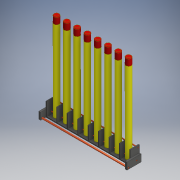
# Autodesk Inventor part: Rampa Lápices 2
Saved by Autodesk Inventor 2016 (Build 200138000, 138)
## iProperties
Created: 2016-06-22
Part Number: Rampa Lápices 2
Material: Generic
Document SubType Name: Modeling
Designer: SCM
Density: 1 g/cm^3
Appearance: Generic
Author: SCM
Autodesk Inventor part; units mm, degrees
ref_plane "YZ Plane" through (0, 0, 0) normal (1, 0, 0) x (0, 1, 0)
sketch "Sketch1" plane through (0, 0, 0) normal (0, 0, 1) x (1, 0, 0)
  line L0 (-120, -20) -> (120, -20)
  line L1 (120, -20) -> (120, 20)
  line L2 (120, 20) -> (-120, 20) construction
  line L3 (-120, 20) -> (-120, -20)
  line L4 (-120, 20) -> (-117.5, 20)
  line L5 (-117.5, 20) -> (-117.5, -17.5)
  line L6 (-117.5, -17.5) -> (117.5, -17.5) construction
  line L7 (117.5, -17.5) -> (117.5, 20)
  line L8 (120, 20) -> (117.5, 20)
  line L9 (-90.3125, -17.5) -> (-87.8125, -17.5) construction
  line L10 (-87.8125, -17.5) -> (-87.8125, 20)
  line L11 (-87.8125, 20) -> (-90.3125, 20)
  line L12 (-90.3125, 20) -> (-90.3125, -17.5)
  line L13 (-60.625, -17.5) -> (-58.125, -17.5) construction
  line L14 (-58.125, -17.5) -> (-58.125, 20)
  line L15 (-58.125, 20) -> (-60.625, 20)
  line L16 (-60.625, 20) -> (-60.625, -17.5)
  line L17 (-30.9375, -17.5) -> (-28.4375, -17.5) construction
  line L18 (-28.4375, -17.5) -> (-28.4375, 20)
  line L19 (-28.4375, 20) -> (-30.9375, 20)
  line L20 (-30.9375, 20) -> (-30.9375, -17.5)
  line L21 (-1.25, -17.5) -> (1.25, -17.5) construction
  line L22 (1.25, -17.5) -> (1.25, 20)
  line L23 (1.25, 20) -> (-1.25, 20)
  line L24 (-1.25, 20) -> (-1.25, -17.5)
  line L25 (28.4375, -17.5) -> (30.9375, -17.5) construction
  line L26 (30.9375, -17.5) -> (30.9375, 20)
  line L27 (30.9375, 20) -> (28.4375, 20)
  line L28 (28.4375, 20) -> (28.4375, -17.5)
  line L29 (58.125, -17.5) -> (60.625, -17.5) construction
  line L30 (60.625, -17.5) -> (60.625, 20)
  line L31 (60.625, 20) -> (58.125, 20)
  line L32 (58.125, 20) -> (58.125, -17.5)
  line L33 (-117.5, -17.5) -> (-90.3125, -17.5)
  line L34 (-87.8125, -17.5) -> (-60.625, -17.5)
  line L35 (-58.125, -17.5) -> (-30.9375, -17.5)
  line L36 (-28.4375, -17.5) -> (-1.25, -17.5)
  line L37 (1.25, -17.5) -> (28.4375, -17.5)
  line L38 (30.9375, -17.5) -> (58.125, -17.5)
  line L39 (60.625, -17.5) -> (91.5625, -17.5) construction
  line L40 (63.125, -17.5) -> (117.5, -17.5) construction
  line L41 (63.125, -17.5) -> (91.5625, -17.5) construction
  line L42 (90.3125, -17.5) -> (87.8125, -17.5) construction
  line L43 (87.8125, -17.5) -> (87.8125, 20)
  line L44 (87.8125, 20) -> (90.3125, 20)
  line L45 (90.3125, 20) -> (90.3125, -17.5)
  line L46 (60.625, -17.5) -> (87.8125, -17.5)
  line L47 (90.3125, -17.5) -> (117.5, -17.5)
  point P0 (0, 0)
  point P1 (120, 0)
  point P2 (0, -20)
  point P3 (94.0625, 20)
  dimension "d2" = 40
  dimension "d3" = 240
  dimension "d4" = 2.5
  dimension "d5" = 2.5
  dimension "d6" = 2.5
  dimension "d7" = 27.1875
  dimension "d8" = 27.1875
  dimension "d9" = 27.1875
  dimension "d10" = 27.1875
  dimension "d11" = 27.1875
  dimension "d12" = 27.1875
  dimension "d24" = 27.1875
  constraints: 92 end point, 15 parallel, 14 horizontal, 12 perpendicular, 10 collinear, 3 midpoint, 3 vertical, 1 horizontal alignment, 1 vertical alignment, 23 other
  measures "d2" distance of L0.end L1.end
  measures "d3" distance of L0.start L0.end
  measures "d4" distance between parallel lines of L3 L5
  measures "d5" distance between parallel lines of L7 L1
  measures "d7" distance between parallel lines of L12 L5
  measures "d8" distance between parallel lines of L16 L10
  measures "d9" distance between parallel lines of L14 L20
  measures "d10" distance between parallel lines of L24 L18
  measures "d11" distance between parallel lines of L28 L22
  measures "d12" distance between parallel lines of L32 L26
  measures "d24" distance of L30.end L43.end
extrude "Extrusion1" add sketch "Sketch1" along normal blind 25
sketch "Sketch4" plane through (120, -20, 0) normal (1, 0, 0) x (0, 0, -1)
  line L0 (0, 0) -> (-40, 0)
  line L1 (-40, 0) -> (-40, 20)
  line L2 (-40, 20) -> (0, 20)
  line L3 (0, 20) -> (0, 0)
  point P0 (0, 20)
  dimension "d25" = 40
  dimension "d26" = 20
  constraints: 8 end point, 2 parallel, 1 horizontal, 1 perpendicular
  measures "d25" distance of L0.start L0.end
  measures "d26" distance of L0.end L1.end
extrude "Extrusion4" add sketch "Sketch4" along normal blind 5
mirror "Mirror2" about plane through (0, 0, 0) normal (1, 0, 0) of "Extrusion4"
sketch "Sketch5" plane through (125, -20, 0) normal (1, 0, 0) x (0, 0, -1)
  line L0 (-40, 0) -> (0, 0) construction
  line L1 (0, 0) -> (0, 20) construction
  line L2 (0, 20) -> (-40, 20) construction
  line L3 (-40, 20) -> (-40, 0) construction
  point P0 (0, 20)
  point P1 (-36, 4)
  dimension "d29" = 4
  dimension "d30" = 4
  measures "d29" distance from line of L0 point (-36, 4)
  measures "d30" distance from line of L3 point (-36, 4)
hole "Hole1" at (125, -16, 36) direction (-1, 0, 0) diameter 4.5 end through all
sketch "Sketch6" plane through (120, 20, 25) normal (1, 0, 0) x (0, 0, -1)
  line L0 (25, -20) -> (25, 0) construction
  line L1 (25, 0) -> (0, 0) construction
  point P0 (25, -20)
  point P1 (21.5, -5)
  dimension "d38" = 3.5
  dimension "d39" = 5
  measures "d38" distance from line of L0 point (21.5, -5)
  measures "d39" distance from line of L1 point (21.5, -5)
hole "Hole2" at (120, 15, 3.5) direction (-1, 0, 0) diameter 3 end through all
sketch "Sketch7" plane through (125, -20, 0) normal (1, 0, 0) x (0, 0, -1)
  line L0 (0, 0) -> (0, 20) construction
  circle A0 centre (-36, 4) radius 2.25 construction
  line L1 (-40, 0) -> (0, 0) construction
  line L2 (0, 0) -> (0, 20) construction
  line L3 (0, 20) -> (-40, 20) construction
  line L4 (-40, 20) -> (-40, 0) construction
  circle A1 centre (-12.5, 10) radius 1.5
  circle A2 centre (-3.5, 35) radius 1.5 construction
  line L5 (-25, 20) -> (0, 20) construction
  line L6 (0, 20) -> (0, 40) construction
  line L7 (0, 40) -> (-25, 40) construction
  line L8 (-25, 20) -> (-25, 40) construction
  point P0 (0, 20)
  dimension "d47" = 12.5
  dimension "d48" = 10
  dimension "d49" = 3
  constraints: 1 centre point
  measures "d47" distance from line of L8 A1.centre
  measures "d48" distance from line of L1 A1.centre
  measures "d49" diameter of A1
extrude "Extrusion5" cut sketch "Sketch7" against normal up to surface (250 mm away)
sketch "Sketch8" plane through (0, 0, 0) normal (1, 0, 0) x (0, 1, 0)
  circle A0 centre (-16, 36) radius 2.25 projected
  point P0 (0, 0)
extrude "Extrusion6" add sketch "Sketch8" along normal mid plane 250 separate body
sketch "Sketch9" plane through (125, -20, 0) normal (1, 0, 0) x (0, 0, -1)
  circle A0 centre (-12.5, 10) radius 1.5 projected
  point P0 (0, 20)
extrude "Extrusion7" add sketch "Sketch9" against normal up to surface (250 mm away) separate body
sketch "Sketch10" plane through (120, 20, 25) normal (1, 0, 0) x (0, 0, -1)
  circle A0 centre (21.5, -5) radius 1.5 projected
  point P0 (25, -20)
extrude "Extrusion8" add sketch "Sketch10" against normal up to surface (240 mm away) separate body
ref_plane "Work Plane1" through (-14.8438, -17.5, 0) normal (1, 0, 0) x (0, 0, -1)
sketch "Sketch11" plane through (-14.8438, -17.5, 0) normal (1, 0, 0) x (0, 0, -1)
  circle A0 centre (-3.5, 32.5) radius 1.5 construction
  circle A1 centre (-12.5, 7.5) radius 1.5 construction
  line L0 (-12.5, 2.5) -> (-5, 2.5)
  line L1 (-5, 2.5) -> (-5, 252.5)
  line L2 (-5, 252.5) -> (-12.5, 252.5)
  line L3 (-12.5, 252.5) -> (-12.5, 2.5)
  point P0 (0, 17.5)
  dimension "d58" = 5
  dimension "d59" = 250
  constraints: 8 end point, 2 parallel, 1 horizontal, 1 perpendicular, 1 point on line, 1 tangent
  measures "d58" distance from line of L0 A1.centre
  measures "d59" distance between parallel lines of L0 L2
revolve "Revolution1" add sketch "Sketch11" angle 360 about axis through (-14.8438, 235, 12.5) along (0, -1, 0) separate body
pattern_linear "Rectangular Pattern1" count 8 spacing 29.1875 along (1, 0, 0) of "Revolution1" first direction both ways yes bodies 5
ref_plane "Work Plane2" through (101.9062, 215, 12.5) normal (0, 1, 0) x (1, 0, 0)
split_face "Split1"
fillet "Fillet1" radius 2 8 edges at (101.9062, 235, 20) (72.7188, 235, 20) (43.5312, 235, 20) (14.3438, 235, 20) (-14.8437, 235, 20) (-44.0312, 235, 20) (-73.2188, 235, 20) (-102.4062, 235, 20)
sketch "Sketch12" plane through (0, 0, 0) normal (1, 0, 0) x (0, 1, 0)
  circle A0 centre (-10, 12.5) radius 1.5 construction
  circle A1 centre (-16, 36) radius 2.25 construction
  line L0 (-20, 40) -> (-20, 0) construction
  line L1 (-20, 0) -> (0, 0) construction
  line L2 (0, 0) -> (0, 40) construction
  line L3 (0, 40) -> (-20, 40) construction
  circle A2 centre (-10, 12.5) radius 1.5 construction
  circle A3 centre (15, 3.5) radius 1.5 construction
  line L4 (20, 0) -> (-17.5, 0) construction
  line L5 (-17.5, 0) -> (-17.5, 25) construction
  line L6 (20, 25) -> (-17.5, 25) construction
  line L7 (20, 0) -> (20, 25) construction
  line L8 (-20, 0) -> (-26, 0)
  line L9 (-26, 0) -> (-26, 15)
  line L10 (-26, 15) -> (-20, 15)
  line L11 (-20, 15) -> (-20, 0)
  point P0 (0, 0)
  point P1 (-20, 25)
  dimension "d69" = 6
  dimension "d70" = 15
  constraints: 8 end point, 2 parallel, 1 horizontal, 1 perpendicular, 1 point on line
  measures "d69" distance of L0.end L8.end
  measures "d70" distance of L8.end L9.end
extrude "Extrusion9" add sketch "Sketch12" along normal mid plane 12.5 bodies 1
sketch "Sketch13" plane through (0, 0, 25) normal (0, 0, 1) x (1, 0, 0)
  line L0 (-120, -20) -> (120, -20) construction
  line L1 (117.5, 20) -> (117.5, -17.5) construction
  line L2 (-117.5, -17.5) -> (-117.5, 20) construction
  line L3 (117.5, -30) -> (-117.5, -30)
  line L4 (-117.5, -30) -> (-117.5, 220)
  line L5 (-117.5, 220) -> (117.5, 220)
  line L6 (117.5, 220) -> (117.5, -30)
  point P0 (0, 0)
  dimension "d71" = 10
  dimension "d72" = 250
  constraints: 8 end point, 2 collinear, 2 parallel, 1 horizontal, 1 perpendicular
  measures "d71" distance between parallel lines of L0 L3
  measures "d72" distance of L5.end L3.start
extrude "Extrusion10" add sketch "Sketch13" along normal blind 250 separate body
equation "\"d5\" = d4"
equation "\"d6\" = d4"
equation "\"d8\" = d7"
equation "\"d9\" = d7"
equation "\"d10\" = d7"
equation "\"d11\" = d7"
equation "\"d12\" = d7"
equation "\"d24\" = d7"
equation "\"d30\" = d29"
equation "\"d47\" = 0.5 * d14"
equation "\"d48\" = 0.5 * d26"
equation "\"d52\" = d3 + 2 * d27"
equation "\"d54\" = d3 + 2 * d27"
equation "\"d56\" = d3 + 2 * d27"
equation "\"d14\" = 25"
equation "\"d27\" = 5"
